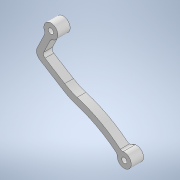
# Autodesk Inventor part: leg_link_3
Saved by Autodesk Inventor 2020 (Build 240168000, 168)
## iProperties
Created: 2020-12-12
Part Number: leg_link_3
Material: Generic
Document SubType Name: Modeling
Designer: Shuang Peng
Density: 1 g/cm^3
Appearance: Default
Author: Shuang Peng
Autodesk Inventor part; units mm, degrees
ref_plane "YZ Plane" through (0, 0, 0) normal (1, 0, 0) x (0, 1, 0)
ref_plane "XZ Plane" through (0, 0, 0) normal (0, 1, 0) x (-1, 0, 0)
ref_plane "XY Plane" through (0, 0, 0) normal (0, 0, 1) x (1, 0, 0)
sketch "Sketch1" plane through (0, 0, 0) normal (0, 0, 1) x (1, 0, 0)
  circle A0 centre (9.329895, 6.999479) radius 4
  line L0 (9.329895, 6.999479) -> (-2.391324, -17.323617)
  circle A1 centre (51.212876, -35.96348) radius 4
  line L1 (9.329895, 6.999479) -> (-2.391324, -17.323617) construction
  line L2 (7.753398, 7.759188) -> (-3.967821, -16.563909)
  line L3 (-0.814827, -18.083326) -> (10.906392, 6.239771)
  arc A2 (10.906392, 6.239771) -> (7.753398, 7.759188) centre (9.329895, 6.999479) ccw
  arc A3 (-3.967821, -16.563909) -> (-0.814827, -18.083326) centre (-2.391324, -17.323617) ccw
  arc A4 (-2.542999, -15.580203) -> (-2.239649, -19.067032) centre (-2.391324, -17.323617) ccw
  arc A5 (49.95979, -37.185067) -> (52.465962, -34.741893) centre (51.212876, -35.96348) ccw
  arc A6 (49.95979, -37.185067) -> (-2.239649, -19.067032) centre (2.770217, -88.887525) ccw
  arc A7 (52.465962, -34.741893) -> (-2.542999, -15.580203) centre (4.022714, -85.271604) ccw
  point P0 (0, 0)
  point P1 (3.469285, -5.162069)
  point P2 (47.351434, -34.919803)
  point P3 (49.725474, -32.250309)
  point P4 (0.497325, -15.360435)
  point P5 (9.34492, 2.999507)
  point P6 (6.191926, 4.518925)
  point P7 (-2.239649, -19.067032)
  dimension "d0" = 8
  dimension "d1" = 27
  dimension "d3" = 8
  dimension "d4" = 3.5
  dimension "d6" = 3.5
  dimension "d7" = 70
  dimension "d8" = 70
  constraints: 12 point on circle, 10 end point, 8 centre point, 4 tangent, 2 coincident, 2 equal length, 1 midpoint, 2 other
  measures "d0" diameter of A0
  measures "d1" distance of L0.start L0.end
  measures "d3" diameter of A1
  measures "d4" diameter of A3
  measures "d6" diameter of A5
  measures "d7" radius of A6
  measures "d8" radius of A7
extrude "Extrusion1" add sketch "Sketch1" along normal blind 7
sketch "Sketch2" plane through (0, 0, 7) normal (0, 0, 1) x (1, 0, 0)
  line L0 (0.497325, -15.360435) -> (9.34492, 2.999507)
  arc A0 (9.34492, 2.999507) -> (6.191926, 4.518925) centre (9.329895, 6.999479) ccw
  line L1 (6.191926, 4.518925) -> (-3.967821, -16.563909)
  arc A1 (-3.967821, -16.563909) -> (-2.239649, -19.067032) centre (-2.391324, -17.323617) ccw
  arc A2 (47.351434, -34.919803) -> (-2.239649, -19.067032) centre (2.770217, -88.887525) ccw
  arc A3 (47.351434, -34.919803) -> (49.725474, -32.250309) centre (51.212876, -35.96348) ccw
  arc A4 (49.725474, -32.250309) -> (0.497325, -15.360435) centre (4.022714, -85.271604) ccw
  point P0 (0, 0)
hole "Hole1" at (51.212876, -35.96348, 7) at (9.329895, 6.999479, 7) direction (0, 0, -1) diameter 3 depth 8
sketch "Sketch3" plane through (0, 0, 0) normal (0, 0, -1) x (-1, 0, 0)
  circle A0 centre (-51.212876, -35.96348) radius 1.5
  circle A1 centre (-9.329895, 6.999479) radius 1.5
  line L0 (-0.497325, -15.360435) -> (-9.34492, 2.999507)
  arc A2 (-0.497325, -15.360435) -> (-49.725474, -32.250309) centre (-4.022714, -85.271604) ccw
  arc A3 (-49.725474, -32.250309) -> (-47.351434, -34.919803) centre (-51.212876, -35.96348) ccw
  arc A4 (2.239649, -19.067032) -> (-47.351434, -34.919803) centre (-2.770217, -88.887525) ccw
  arc A5 (2.239649, -19.067032) -> (3.967821, -16.563909) centre (2.391324, -17.323617) ccw
  line L1 (-6.191926, 4.518925) -> (3.967821, -16.563909)
  arc A6 (-6.191926, 4.518925) -> (-9.34492, 2.999507) centre (-9.329895, 6.999479) ccw
  circle A7 centre (-9.329895, 6.999479) radius 4
  circle A8 centre (-51.212876, -35.96348) radius 4
  point P0 (0, 0)
  point P1 (-49.725474, -32.250309)
  dimension "d18" = 8
  dimension "d19" = 8
  constraints: 2 centre point, 2 coincident
  measures "d18" diameter of A7
  measures "d19" diameter of A8
extrude "Extrusion2" cut sketch "Sketch3" against normal blind 2 contours L0 A7 L1 A5 A4 A8 A2
fillet "Fillet1" radius 2 6 edges at (47.3514, -34.9198, 4.5) (48.2239, -33.3053, 2) (49.7255, -32.2503, 4.5) (9.3449, 2.9995, 4.5) (7.5934, 3.3961, 2) (6.1919, 4.5189, 4.5)
fillet "Fillet2" radius 1 1 edges at (0.4973, -15.3604, 4.5)
body "Solid1"
